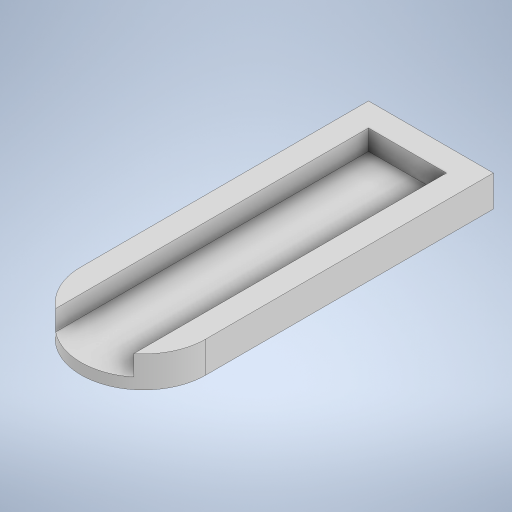
# Autodesk Inventor part: Tapa1
Saved by Autodesk Inventor 2024 (Build 280153000, 153)
## iProperties
Created: 2024-04-28
Part Number: Tapa1
Material: Generic
Document SubType Name: Modeling
Designer: samue
Density: 1 g/cm^3
Appearance: Default
Author: samue
Autodesk Inventor part; units mm, degrees
ref_plane "YZ Plane" through (0, 0, 0) normal (1, 0, 0) x (0, 1, 0)
ref_plane "XZ Plane" through (0, 0, 0) normal (0, 1, 0) x (-1, 0, 0)
ref_plane "XY Plane" through (0, 0, 0) normal (0, 0, 1) x (1, 0, 0)
sketch "Sketch1" plane through (0, 0, 0) normal (0, 1, 0) x (-1, 0, 0)
  arc A0 (4, 0) -> (-4, 0) centre (0, 0) ccw
  line L0 (4, 0) -> (4, -18.4143)
  line L1 (4, -18.4143) -> (-4, -18.4143)
  line L2 (-4, -18.4143) -> (-4, 0)
  line L3 (2.5, -16.9143) -> (2.5, 0)
  arc A1 (2.5, 0) -> (-2.5, 0) centre (0, 0) ccw
  line L4 (-2.5, 0) -> (-2.5, -16.9143)
  line L5 (-2.5, -16.9143) -> (2.5, -16.9143)
  dimension "d0" = 8
  dimension "d3" = 1.5
  constraints: 12 end point, 4 point on circle, 2 centre point, 2 vertical, 1 coincident, 1 horizontal, 3 other
  measures "d0" diameter of A0
  measures "d3" distance between parallel lines of L0 L3
extrude "Extrusion2" add sketch "Sketch1" along normal blind 2
extrude "Extrusion3" add sketch "Sketch1" along normal blind 1 contours L5 L4 A1 L3
sketch "Sketch2" plane through (4, 0, -18.4143) normal (0, 0, -1) x (-1, 0, 0)
  line L0 (0, 0) -> (8, 0) projected
  line L1 (1.5, 2) -> (6.5, 2) projected
  line L2 (2, 2) -> (6, 2)
  line L3 (2, 2) -> (2, 0.3)
  line L4 (2, 0.3) -> (6, 0.3)
  line L5 (6, 0.3) -> (6, 2)
  point P0 (4, 2)
  point P1 (4, 0)
  dimension "d11" = 4
  dimension "d12" = 1.7
  constraints: 8 end point, 2 midpoint, 2 perpendicular, 1 collinear, 1 point on line, 1 vertical, 1 vertical alignment
  measures "d11" distance of L2.start L2.end
  measures "d12" distance of L2.start L3.end
sketch "Sketch3" plane through (-2.5, 2, -16.9143) normal (0, 0, 1) x (1, 0, 0)
  line L0 (0.5, -1.7) -> (0.5, 0) projected
  line L1 (6.5, 0) -> (-1.5, 0) projected
  line L2 (4.5, -1.7) -> (0.5, -1.7) projected
  line L3 (4.5, 0) -> (4.5, -1.7) projected
  line L4 (5, -1) -> (5, 0) projected
  line L5 (5, -1) -> (5, 0) projected
  line L6 (0, 0) -> (5, 0) projected
  line L7 (0, -1) -> (5, -1) projected
  line L8 (0, -1) -> (5, -1) projected
  line L9 (5, -1) -> (5, 0) projected
  line L10 (0, 0) -> (5, 0) projected
  line L11 (0, -1) -> (0, 0) projected
  line L12 (5, -1) -> (0, -1) projected
  line L13 (0, -1) -> (5, -1) projected
  line L14 (-1.5, 0) -> (6.5, 0) projected
  line L15 (6.5, 0) -> (-1.5, 0) projected
  line L16 (0, 0) -> (5, 0) projected
  line L17 (5, 0) -> (0, 0) projected
  line L18 (6.5, -2) -> (-1.5, -2) projected
  line L19 (-1.5, -2) -> (-1.5, 0) projected
  line L20 (6.5, 0) -> (-1.5, 0) projected
  line L21 (6.5, -2) -> (6.5, 0) projected
  line L22 (5, 0) -> (0, 0) projected
  line L23 (4.5, 0) -> (0.5, 0) projected
  point P0 (2.5, -2)
  point P1 (2.5, 0)
  constraints: 3 other
extrude "Extrusion4" cut sketch "Sketch3" along normal blind 22 contours L7 L11 L1 L0 | L0 L1 L3 L7 | L3 L1 L4 L7
sketch "Sketch4" plane through (0, 1, 0) normal (0, 1, 0) x (1, 0, 0)
  line L0 (-2.5, 16.9143) -> (2.5, 16.9143) projected
  line L1 (2.5, 16.9143) -> (-2.5, 16.9143)
  line L2 (-2.5, 16.9143) -> (-2.5, -4.1065)
  line L3 (-2.5, -4.1065) -> (2.5, -4.1065)
  line L4 (2.5, -4.1065) -> (2.5, 16.9143)
  point P0 (0, 0)
  constraints: 8 end point, 2 parallel, 1 horizontal, 1 perpendicular
extrude "Extrusion5" cut sketch "Sketch4" against normal blind 0.3
body "Solid2"
